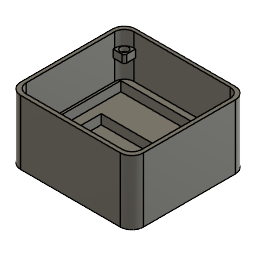
box_pcb_final (Autodesk Fusion 360 design; units mm, degrees)
part number: 2025-11-23-22-43-50-638
Autodesk Fusion 360 part; units mm, degrees
sketch "Sketch1" plane through (0, 0, 0) normal (0, 1, 0) x (1, 0, 0)
  line L0 (16.51, 76.2) -> (80.01, 76.2)
  line L1 (86.36, 69.85) -> (86.36, 11.43)
  line L2 (80.01, 5.08) -> (16.51, 5.08)
  line L3 (10.16, 11.43) -> (10.16, 69.85)
  arc A0 (16.51, 76.2) -> (10.16, 69.85) centre (16.51, 69.85) ccw
  arc A1 (86.36, 69.85) -> (80.01, 76.2) centre (80.01, 69.85) ccw
  arc A2 (80.01, 5.08) -> (86.36, 11.43) centre (80.01, 11.43) ccw
  arc A3 (10.16, 11.43) -> (16.51, 5.08) centre (16.51, 11.43) ccw
  point P0 (10.16, 76.2)
  point P1 (86.36, 76.2)
  point P2 (10.16, 5.08)
  dimension "d1" = 76.2
  dimension "d2" = 71.12
  dimension "d3" = 6.35
  constraint horizontal L0
  constraint vertical L1
  constraint horizontal L2
  constraint vertical L3
  constraint coincident P0 L0
  constraint coincident P0 L3
  constraint tangent L0 A0
  constraint tangent L3 A0
  constraint coincident P1 L0
  constraint coincident P1 L1
  constraint tangent L0 A1
  constraint tangent L1 A1
  constraint equal A0 A1
  constraint tangent L1 A2
  constraint tangent L2 A2
  constraint equal A0 A2
  constraint coincident P2 L2
  constraint coincident P2 L3
  constraint tangent L2 A3
  constraint tangent L3 A3
  constraint equal A0 A3
  measures "d1" distance of P0 P1
  measures "d2" distance of P0 P2
  measures "d3" radius of A0
extrude "Extrude1" add sketch "Sketch1" along normal blind 15.875 makes body 1
sketch "Sketch2" plane through (0, 15.875, 0) normal (0, 1, 0) x (-1, 0, 0)
  arc A0 (-16.51, -76.2) -> (-10.16, -69.85) centre (-16.51, -69.85) ccw
  line L0 (-10.16, -69.85) -> (-10.16, -11.43)
  arc A1 (-10.16, -11.43) -> (-16.51, -5.08) centre (-16.51, -11.43) ccw
  line L1 (-16.51, -5.08) -> (-80.01, -5.08)
  arc A2 (-80.01, -5.08) -> (-86.36, -11.43) centre (-80.01, -11.43) ccw
  line L2 (-86.36, -11.43) -> (-86.36, -69.85)
  arc A3 (-86.36, -69.85) -> (-80.01, -76.2) centre (-80.01, -69.85) ccw
  line L3 (-80.01, -76.2) -> (-16.51, -76.2)
  line L4 (-17.78, -53.34) -> (-80.01, -53.34)
  line L5 (-80.01, -53.34) -> (-80.01, -12.192)
  line L6 (-80.01, -12.192) -> (-17.78, -12.192)
  line L7 (-17.78, -12.192) -> (-17.78, -53.34)
  dimension "d6" = 62.23
  dimension "d7" = 41.148
  constraint horizontal L4
  constraint vertical L5
  constraint horizontal L6
  constraint vertical L7
  measures "d6" distance of L4.start L4.end
  measures "d7" distance of L4.start L6.end
extrude "Extrude2" cut sketch "Sketch2" against normal blind 12.7 contours L4 L5 L6 L7 bodies 1
sketch "Sketch3" plane through (0, 15.875, 0) normal (0, 1, 0) x (-1, 0, 0)
  line L0 (-80.01, -53.34) -> (-80.01, -12.192)
  line L1 (-80.01, -12.192) -> (-17.78, -12.192)
  line L2 (-17.78, -12.192) -> (-17.78, -53.34)
  line L3 (-17.78, -53.34) -> (-80.01, -53.34)
  arc A0 (-16.51, -76.2) -> (-10.16, -69.85) centre (-16.51, -69.85) ccw
  line L4 (-10.16, -69.85) -> (-10.16, -11.43)
  arc A1 (-10.16, -11.43) -> (-16.51, -5.08) centre (-16.51, -11.43) ccw
  line L5 (-16.51, -5.08) -> (-80.01, -5.08)
  arc A2 (-80.01, -5.08) -> (-86.36, -11.43) centre (-80.01, -11.43) ccw
  line L6 (-86.36, -11.43) -> (-86.36, -69.85)
  arc A3 (-86.36, -69.85) -> (-80.01, -76.2) centre (-80.01, -69.85) ccw
  line L7 (-80.01, -76.2) -> (-16.51, -76.2)
  line L8 (-12.694, -72.3484) -> (-83.814, -72.3484)
  line L9 (-83.814, -72.3484) -> (-83.814, -8.8484)
  line L10 (-83.814, -8.8484) -> (-12.694, -8.8484)
  line L11 (-12.694, -8.8484) -> (-12.694, -72.3484)
  dimension "d10" = 71.12
  dimension "d11" = 63.5
  constraint horizontal L8
  constraint vertical L9
  constraint horizontal L10
  constraint vertical L11
  measures "d10" distance of L8.start L8.end
  measures "d11" distance of L8.start L10.end
extrude "Extrude3" cut sketch "Sketch3" against normal blind 6.35 contours L8 L9 L10 L11 bodies 1
sketch "Sketch4" plane through (0, 15.875, 0) normal (0, 1, 0) x (-1, 0, 0)
  line L0 (-83.814, -72.3484) -> (-83.814, -8.8484)
  line L1 (-83.814, -8.8484) -> (-12.694, -8.8484)
  line L2 (-12.694, -8.8484) -> (-12.694, -72.3484)
  line L3 (-12.694, -72.3484) -> (-83.814, -72.3484)
  arc A0 (-16.51, -76.2) -> (-10.16, -69.85) centre (-16.51, -69.85) ccw
  line L4 (-10.16, -69.85) -> (-10.16, -11.43)
  arc A1 (-10.16, -11.43) -> (-16.51, -5.08) centre (-16.51, -11.43) ccw
  line L5 (-16.51, -5.08) -> (-80.01, -5.08)
  arc A2 (-80.01, -5.08) -> (-86.36, -11.43) centre (-80.01, -11.43) ccw
  line L6 (-86.36, -11.43) -> (-86.36, -69.85)
  arc A3 (-86.36, -69.85) -> (-80.01, -76.2) centre (-80.01, -69.85) ccw
  line L7 (-80.01, -76.2) -> (-16.51, -76.2)
  line L8 (-15.4725, -77.1132) -> (-81.2585, -77.1132)
  line L9 (-87.6085, -70.7632) -> (-87.6085, -10.0572)
  line L10 (-81.2585, -3.7072) -> (-15.4725, -3.7072)
  line L11 (-9.1225, -10.0572) -> (-9.1225, -70.7632)
  arc A4 (-15.4725, -77.1132) -> (-9.1225, -70.7632) centre (-15.4725, -70.7632) ccw
  arc A5 (-87.6085, -70.7632) -> (-81.2585, -77.1132) centre (-81.2585, -70.7632) ccw
  arc A6 (-81.2585, -3.7072) -> (-87.6085, -10.0572) centre (-81.2585, -10.0572) ccw
  arc A7 (-9.1225, -10.0572) -> (-15.4725, -3.7072) centre (-15.4725, -10.0572) ccw
  point P0 (-9.1225, -77.1132)
  point P1 (-87.6085, -77.1132)
  point P2 (-9.1225, -3.7072)
  dimension "d14" = 78.486
  dimension "d15" = 73.406
  dimension "d16" = 6.35
  constraint horizontal L8
  constraint vertical L9
  constraint horizontal L10
  constraint vertical L11
  constraint coincident P0 L8
  constraint coincident P0 L11
  constraint tangent L8 A4
  constraint tangent L11 A4
  constraint coincident P1 L8
  constraint coincident P1 L9
  constraint tangent L8 A5
  constraint tangent L9 A5
  constraint equal A4 A5
  constraint tangent L9 A6
  constraint tangent L10 A6
  constraint equal A4 A6
  constraint coincident P2 L11
  constraint coincident P2 L10
  constraint tangent L11 A7
  constraint tangent L10 A7
  constraint equal A4 A7
  measures "d14" distance of P0 P1
  measures "d15" distance of P0 P2
  measures "d16" radius of A4
extrude "Extrude4" add sketch "Sketch4" along normal blind 25.4 separate body contours L8 L9 L10 L11 A4 A5 A6 A7 makes body 2
extrude "Extrude5" add 1 faces at (58.9136, 15.875, -4.1648) along direction (0, -1, 0) blind 15.24 on bodies 2 bodies 1 2
sketch "Sketch5" plane through (0, 15.875, 0) normal (0, 1, 0) x (-1, 0, 0)
  line L0 (-83.814, -72.3484) -> (-83.814, -8.8484)
  line L1 (-83.814, -8.8484) -> (-12.694, -8.8484)
  line L2 (-12.694, -8.8484) -> (-12.694, -72.3484)
  line L3 (-12.694, -72.3484) -> (-83.814, -72.3484)
  arc A0 (-16.51, -76.2) -> (-10.16, -69.85) centre (-16.51, -69.85) ccw
  line L4 (-10.16, -69.85) -> (-10.16, -11.43)
  arc A1 (-10.16, -11.43) -> (-16.51, -5.08) centre (-16.51, -11.43) ccw
  line L5 (-16.51, -5.08) -> (-80.01, -5.08)
  arc A2 (-80.01, -5.08) -> (-86.36, -11.43) centre (-80.01, -11.43) ccw
  line L6 (-86.36, -11.43) -> (-86.36, -69.85)
  arc A3 (-86.36, -69.85) -> (-80.01, -76.2) centre (-80.01, -69.85) ccw
  line L7 (-80.01, -76.2) -> (-16.51, -76.2)
  line L8 (-60.1908, -74.691) -> (-62.6165, -74.691)
  line L9 (-62.6165, -74.691) -> (-62.6165, -72.2653)
  line L10 (-62.6165, -72.2653) -> (-60.1908, -72.2653)
  line L11 (-60.1908, -72.2653) -> (-60.1908, -74.691)
  dimension "d21" = 2.4257
  dimension "d22" = 2.4257
  constraint horizontal L8
  constraint vertical L9
  constraint horizontal L10
  constraint vertical L11
  measures "d21" distance of L8.start L8.end
  measures "d22" distance of L8.start L10.end
extrude "Extrude6" cut sketch "Sketch5" against normal blind 6.35 contours L3 L8 L9 L11 bodies 1
sketch "Sketch6" plane through (0, 9.525, 0) normal (0, 1, 0) x (-1, 0, 0)
  line L0 (-17.78, -12.192) -> (-17.78, -53.34)
  line L1 (-17.78, -53.34) -> (-80.01, -53.34)
  line L2 (-80.01, -53.34) -> (-80.01, -12.192)
  line L3 (-80.01, -12.192) -> (-17.78, -12.192)
  line L4 (-12.694, -8.8484) -> (-83.814, -8.8484)
  line L5 (-83.814, -8.8484) -> (-83.814, -72.3484)
  line L6 (-83.814, -72.3484) -> (-62.6165, -72.3484)
  line L7 (-62.6165, -72.3484) -> (-62.6165, -74.691)
  line L8 (-62.6165, -74.691) -> (-60.1908, -74.691)
  line L9 (-60.1908, -74.691) -> (-60.1908, -72.3484)
  line L10 (-60.1908, -72.3484) -> (-12.694, -72.3484)
  line L11 (-12.694, -72.3484) -> (-12.694, -8.8484)
  line L12 (-80.01, -30.5129) -> (-83.814, -30.5129)
  line L13 (-83.814, -30.5129) -> (-83.814, -33.1045)
  line L14 (-83.814, -33.1045) -> (-80.01, -33.1045)
  line L15 (-80.01, -33.1045) -> (-80.01, -30.5129)
  line L16 (-83.814, -33.1045) -> (-84.0211, -33.1045)
  line L17 (-84.0211, -33.1045) -> (-84.0211, -30.5645)
  line L18 (-84.0211, -30.5645) -> (-83.814, -30.5645)
  line L19 (-83.814, -30.5645) -> (-83.814, -33.1045)
  dimension "d29" = 2.54
  constraint horizontal L12
  constraint vertical L13
  constraint horizontal L14
  constraint vertical L15
  constraint coincident L5 L13.end
  constraint coincident L2 L12.start
  constraint horizontal L16
  constraint vertical L17
  constraint horizontal L18
  constraint vertical L19
  measures "d29" distance of L13.end L18.end
extrude "Extrude7" cut 1 faces at (60.1073, 13.7583, -8.8484) along direction (0, 0, 1) blind 1.016 on bodies 1 bodies 1
extrude "Extrude8" cut 1 faces at (12.694, 13.7583, -29.3377) along direction (-1, 0, 0) blind 1.016 on bodies 1 bodies 1
extrude "Extrude9" cut sketch "Sketch6" against normal blind 6.35 contours L2 L5 L12 L13 L14 L15 L19 bodies 1
sketch "Sketch7" plane through (83.814, 0, 0) normal (-1, 0, 0) x (0, 0, 1)
  line L0 (-7.8324, 15.875) -> (-72.3484, 15.875)
  line L1 (-72.3484, 15.875) -> (-72.3484, 9.525)
  line L2 (-72.3484, 9.525) -> (-33.1045, 9.525)
  line L3 (-33.1045, 9.525) -> (-33.1045, 3.175)
  line L4 (-33.1045, 3.175) -> (-30.5129, 3.175)
  line L5 (-30.5129, 3.175) -> (-30.5129, 9.525)
  line L6 (-30.5129, 9.525) -> (-7.8324, 9.525)
  line L7 (-7.8324, 9.525) -> (-7.8324, 15.875)
  line L8 (-33.0815, 15.875) -> (-30.5415, 15.875)
  line L9 (-30.5415, 15.875) -> (-30.5415, 3.182)
  line L10 (-30.5415, 3.182) -> (-33.0815, 3.182)
  line L11 (-33.0815, 3.182) -> (-33.0815, 15.875)
  dimension "d32" = 2.54
  constraint horizontal L8
  constraint vertical L9
  constraint horizontal L10
  constraint vertical L11
  constraint coincident L0 L8.start
  measures "d32" distance of L8.start L8.end
extrude "Extrude10" cut sketch "Sketch7" against normal blind 2.54 contours L0 L8 L9 L10 L11 bodies 1
extrude "Extrude11" add 1 faces at (60.9994, 13.7583, -74.691) along direction (0, 0, 1) blind 2.3368 on bodies 1 bodies 1
ref_plane "WorkPlane1" through (48.3655, 33.655, -40.4102) normal (0, 1, 0) x (-1, 0, 0)
sketch "Sketch8" plane through (0, 33.655, 0) normal (0, 1, 0) x (1, 0, 0)
ref_plane "WorkPlane2" through (48.3655, 34.925, -40.4102) normal (0, 1, 0) x (-1, 0, 0)
sketch "Sketch9" plane through (0, 34.925, 0) normal (0, 1, 0) x (1, 0, 0)
  arc A0 (16.51, 76.2) -> (10.16, 69.85) centre (16.51, 69.85) ccw
  line L0 (10.16, 69.85) -> (10.16, 11.43)
  arc A1 (10.16, 11.43) -> (16.51, 5.08) centre (16.51, 11.43) ccw
  line L1 (16.51, 5.08) -> (80.01, 5.08)
  arc A2 (80.01, 5.08) -> (86.36, 11.43) centre (80.01, 11.43) ccw
  line L2 (86.36, 11.43) -> (86.36, 69.85)
  arc A3 (86.36, 69.85) -> (80.01, 76.2) centre (80.01, 69.85) ccw
  line L3 (80.01, 76.2) -> (16.51, 76.2)
  line L4 (16.51, 5.08) -> (16.51, 11.43)
  line L5 (16.51, 11.43) -> (10.16, 11.43)
  arc A4 (80.01, 5.08) -> (86.36, 11.43) centre (80.01, 11.43) ccw
  line L6 (80.01, 5.08) -> (80.01, 11.43)
  line L7 (80.01, 11.43) -> (86.36, 11.43)
  arc A5 (10.16, 11.43) -> (16.51, 5.08) centre (16.51, 11.43) ccw
  line L8 (16.51, 69.85) -> (16.51, 76.2)
  line L9 (10.16, 69.85) -> (16.51, 69.85)
  line L10 (80.01, 76.2) -> (80.01, 69.85)
  line L11 (80.01, 69.85) -> (86.36, 69.85)
  line L12 (48.26, 5.08) -> (47.5041, 76.2) construction
  constraint coincident A1.end L1.start
  constraint coincident A1.centre L4.end
  constraint coincident L0.end A1.start
  constraint coincident A2.end L2.start
  constraint coincident L1.end A2.start
  constraint coincident A2.centre A4.centre
  constraint perpendicular L1 L6
  constraint coincident A0.centre L8.start
  constraint coincident A0.start L3.end
  constraint coincident A0.end L0.start
  constraint coincident A3.end L3.start
  constraint coincident A3.centre L10.end
  constraint coincident L2.end A3.start
  constraint midpoint L1 L12.start
  constraint coincident L3 L12.end
extrude "Extrude12" add sketch "Sketch9" against normal blind 5.08 contours A0 L8 L9 | A3 L10 L11 | A1 L4 L5 A5 | A2 A4 L6 L7 bodies 1
move_face "OffsetFaces1" offset 1.016 8 faces at (16.51, 33.2317, -71.9667) (12.2767, 33.2317, -69.85) (82.1267, 33.2317, -69.85) (80.01, 33.2317, -74.0833) (14.3933, 33.2317, -11.43) (16.51, 33.2317, -7.1967) (82.1267, 33.2317, -11.43) (80.01, 31.5383, -9.3133) on bodies 1
fillet "Fillet1" radius 1.524 1 edges at (78.994, 32.385, -12.446) on bodies 1
fillet "Fillet2" radius 1.524 1 edges at (17.526, 32.385, -12.446) on bodies 1
fillet "Fillet3" radius 1.524 1 edges at (78.994, 32.385, -68.834) on bodies 1
fillet "Fillet4" radius 1.524 1 edges at (17.526, 32.385, -68.834) on bodies 1
sketch "Sketch14" plane through (0, 34.925, 0) normal (0, 1, 0) x (-1, 0, 0)
  arc A0 (-80.518, -12.446) -> (-78.994, -10.922) centre (-80.518, -10.922) ccw
  line L0 (-78.994, -10.922) -> (-78.994, -5.08)
  line L1 (-78.994, -5.08) -> (-80.01, -5.08)
  arc A1 (-80.01, -5.08) -> (-86.36, -11.43) centre (-80.01, -11.43) ccw
  line L2 (-86.36, -11.43) -> (-86.36, -12.446)
  line L3 (-86.36, -12.446) -> (-80.518, -12.446)
  circle A2 centre (-82.3098, -9.0797) radius 2.667
  circle A3 centre (-14.1575, -8.9323) radius 2.667
  circle A4 centre (-82.694, -72.0902) radius 2.667
  circle A5 centre (-13.97, -72.39) radius 2.667
  dimension "d60" = 5.334
  dimension "d61" = 5.334
  dimension "d62" = 5.334
  dimension "d63" = 5.334
  measures "d60" diameter of A2
  measures "d61" diameter of A3
  measures "d62" diameter of A4
  measures "d63" diameter of A5
extrude "Extrude14" cut sketch "Sketch14" against normal blind 3.175 contours A2 | A3 | A4 | A5 bodies 1
move_face "OffsetFaces2" offset 1.27 8 faces at (59.3298, 27.7283, -77.1132) (87.1536, 27.7283, -73.1232) (87.6085, 27.7283, -30.2925) (86.9026, 27.7283, -7.1474) (59.3298, 14.1817, -3.7072) (10.2999, 27.7283, -6.3738) (9.1225, 27.7283, -50.5279) (10.8767, 27.7283, -75.1452) on bodies 1
extrude "Extrude15" add 1 faces at (58.9136, 41.275, -3.3181) along direction (0, 1, 0) blind 3.048 on bodies 1 bodies 1
extrude "Extrude16" cut 1 faces at (58.8433, 0, -28.7867) along direction (0, 1, 0) blind 0.635 on bodies 1 bodies 1
sketch "Sketch15" plane through (0, 0.635, 0) normal (0, -1, 0) x (1, 0, 0)
  arc A0 (7.8525, -70.7632) -> (15.4725, -78.3832) centre (15.4725, -70.7632) ccw
  line L0 (15.4725, -78.3832) -> (81.2585, -78.3832)
  arc A1 (81.2585, -78.3832) -> (88.8785, -70.7632) centre (81.2585, -70.7632) ccw
  line L1 (88.8785, -70.7632) -> (88.8785, -10.0572)
  arc A2 (88.8785, -10.0572) -> (81.2585, -2.4372) centre (81.2585, -10.0572) ccw
  line L2 (81.2585, -2.4372) -> (15.4725, -2.4372)
  arc A3 (15.4725, -2.4372) -> (7.8525, -10.0572) centre (15.4725, -10.0572) ccw
  line L3 (7.8525, -10.0572) -> (7.8525, -70.7632)
  line L4 (10.1981, -27.1725) -> (85.8393, -27.1725)
  line L5 (85.8393, -27.1725) -> (85.8393, -52.5725)
  line L6 (85.8393, -52.5725) -> (10.1981, -52.5725)
  line L7 (10.1981, -52.5725) -> (10.1981, -27.1725)
  dimension "d71" = 75.6412
  dimension "d72" = 25.4
  constraint horizontal L4
  constraint vertical L5
  constraint horizontal L6
  constraint vertical L7
  measures "d71" distance of L4.start L4.end
  measures "d72" distance of L4.start L6.end
other "Base Mesh Feature1"
other "Modify1"
other "Modify2"
sketch "Sketch21" plane through (0, 9.525, 0) normal (0, 1, 0) x (-1, 0, 0)
  line L0 (-62.6165, -72.3542) -> (-60.1908, -72.3542)
  line L1 (-60.1908, -72.3542) -> (-60.1908, -72.3484)
  line L2 (-60.1908, -72.3484) -> (-11.678, -72.3484)
  line L3 (-11.678, -72.3484) -> (-11.678, -7.8324)
  line L4 (-11.678, -7.8324) -> (-83.814, -7.8324)
  line L5 (-83.814, -7.8324) -> (-83.814, -30.5129)
  line L6 (-83.814, -30.5129) -> (-80.01, -30.5129)
  line L7 (-80.01, -30.5129) -> (-80.01, -12.192)
  line L8 (-80.01, -12.192) -> (-17.78, -12.192)
  line L9 (-17.78, -12.192) -> (-17.78, -53.34)
  line L10 (-17.78, -53.34) -> (-80.01, -53.34)
  line L11 (-80.01, -53.34) -> (-80.01, -33.1045)
  line L12 (-80.01, -33.1045) -> (-83.814, -33.1045)
  line L13 (-83.814, -33.1045) -> (-83.814, -72.3484)
  line L14 (-83.814, -72.3484) -> (-62.6165, -72.3484)
  line L15 (-62.6165, -72.3484) -> (-62.6165, -72.3542)
  line L16 (-80.01, -30.5129) -> (-83.814, -30.5129)
  line L17 (-83.814, -30.5129) -> (-83.814, -12.2678)
  line L18 (-83.814, -12.2678) -> (-80.01, -12.2678)
  line L19 (-80.01, -12.2678) -> (-80.01, -30.5129)
  constraint horizontal L16
  constraint vertical L17
  constraint horizontal L18
  constraint vertical L19
  constraint coincident L5 L17.end
  constraint coincident L6.end L7.start
extrude "Extrude20" cut sketch "Sketch21" against normal blind 6.35 contours L5 L6 L7 L16 L17 L18 L19 bodies 1
move_face "OffsetFaces3" offset -19.05 1 faces at (84.6607, 11.644, -30.5415) on bodies 1
move_face "OffsetFaces4" offset -1.27 1 faces at (37.4011, 0.635, -53.0679) on bodies 1
